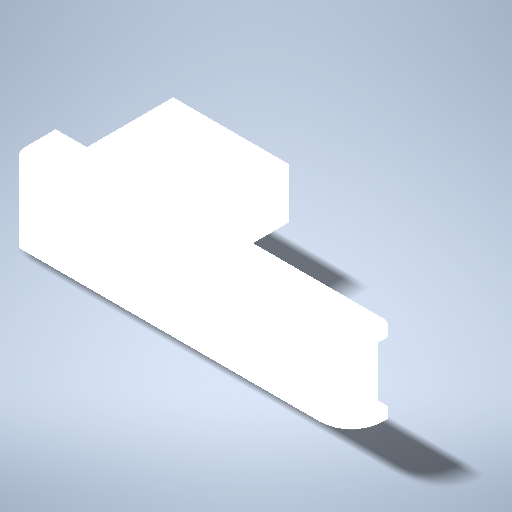
# Autodesk Inventor part: stereotax_holder_side
Saved by Autodesk Inventor 2025 (Build 290162000, 162)
## iProperties
Created: 2023-10-03
Part Number: stereotax_holder_side
Material: Generic
Document SubType Name: Modeling
Designer: mmelin
Density: 1 g/cm^3
Appearance: Default
Author: mmelin
Autodesk Inventor part; units mm, degrees
ref_plane "YZ Plane" through (0, 0, 0) normal (1, 0, 0) x (0, 1, 0)
ref_plane "XZ Plane" through (0, 0, 0) normal (0, 1, 0) x (-1, 0, 0)
ref_plane "XY Plane" through (0, 0, 0) normal (0, 0, 1) x (1, 0, 0)
sketch "Sketch1" plane through (0, 0, 0) normal (0, 0, 1) x (1, 0, 0)
  line L0 (-6.6, -4.4) -> (-23.2373, -4.4) projected
  line L1 (-23.2373, 1) -> (-6.6, 1) projected
  line L2 (-4.6226, -4.4) -> (-25.2226, -4.4)
  line L3 (-25.2226, -4.4) -> (-25.2226, 1)
  line L4 (-25.2226, 1) -> (-4.6226, 1)
  line L5 (-4.6226, 1) -> (-4.6226, -4.4)
  line L6 (-11.6, -0.9) -> (-11.6, -3.4) projected
  line L7 (-4.6226, 0.16) -> (-4.6226, -3.56) projected
  line L8 (-4.6226, 0.16) -> (-15, 0.16) projected
  line L9 (-15, 0.16) -> (-15, -3.56) projected
  line L10 (-15, -3.56) -> (-4.6226, -3.56) projected
  point P0 (0, 0)
  dimension "d1" = 20.6
  dimension "d36" = 0
  constraints: 8 end point, 2 collinear, 2 parallel, 1 horizontal, 1 perpendicular
  measures "d1" distance between parallel lines of L3 L5
  measures "d36" distance between parallel lines of L7 L5
extrude "Extrusion1" add sketch "Sketch1" along normal blind 1.7
sketch "Sketch2" plane through (0, 0, 0) normal (0, 0, -1) x (-1, 0, 0)
  line L0 (4.6226, 0.16) -> (4.6226, -3.56) projected
  line L1 (4.6226, 0.16) -> (15, 0.16) projected
  line L2 (15, 0.16) -> (15, -3.56) projected
  line L3 (15, -3.56) -> (4.6226, -3.56) projected
  line L4 (25.2226, -4.4) -> (4.6226, -4.4) projected
  line L5 (25.2226, 1) -> (25.2226, -4.4) projected
  line L6 (8.5501, -0.0891) -> (8.5501, -3.1391) projected
  line L7 (25.2226, -4.4) -> (4.6226, -4.4) projected
  line L8 (4.6226, -4.4) -> (4.6226, 1) projected
  line L9 (4.6226, 1) -> (25.2226, 1) projected
  line L10 (25.2226, 1) -> (25.2226, -4.4) projected
  line L11 (11.8, -2.35) -> (15, -2.35) projected
  line L12 (11.8, -1.05) -> (11.8, -2.35) projected
  line L13 (15, -1.05) -> (11.8, -1.05) projected
  point P0 (0, 0)
extrude "Extrusion2" add sketch "Sketch2" along normal blind 0.6 contours L8 L9 L5 L4 L3 L2 L1 | L2 L11 L12 L13
fillet "Fillet1" radius 2 1 edges at (-4.6226, -1.7, 1.7)
sketch "Sketch4" plane through (0, 0, -0.6) normal (0, 0, -1) x (-1, 0, 0)
  line L0 (24.45, -3.25) -> (17.25, -3.25)
  line L1 (17.25, -3.25) -> (17.25, -0.15)
  line L2 (17.25, -0.15) -> (24.45, -0.15)
  line L3 (24.45, -0.15) -> (24.45, -3.25)
  line L4 (24.6, -3.4) -> (24.6, 0) projected
  line L5 (17.1, -3.4) -> (24.6, -3.4) projected
  line L6 (17.1, 0) -> (17.1, -3.4) projected
  line L7 (24.6, 0) -> (17.1, 0) projected
  circle A0 centre (20.85, -1.7) radius 1.1 projected
  circle A1 centre (20.85, -1.7) radius 1.1
  point P0 (0, 0)
  dimension "d14" = 0.15
  dimension "d15" = 0.15
  dimension "d16" = 0.15
  dimension "d17" = 0.15
  constraints: 8 end point, 2 parallel, 1 centre point, 1 coincident, 1 concentric, 1 horizontal, 1 perpendicular
  measures "d14" distance between parallel lines of L7 L2
  measures "d15" distance between parallel lines of L6 L1
  measures "d16" distance between parallel lines of L4 L3
  measures "d17" distance between parallel lines of L5 L0
extrude "Extrusion5" add sketch "Sketch4" along normal blind 6.5 contours L0 L1 L2 L3
sketch "Sketch6" plane through (0, 0, 1.7) normal (0, 0, 1) x (1, 0, 0)
  circle A0 centre (-20.85, -1.7) radius 1.1 projected
  circle A1 centre (-20.85, -1.7) radius 1.1
  point P0 (0, 0)
  constraints: 1 centre point, 1 coincident
extrude "Extrusion7" cut sketch "Sketch6" against normal up to surface (8.8 mm away)
sketch "Sketch7" plane through (0, 0, 1.7) normal (0, 0, 1) x (1, 0, 0)
  circle A0 centre (-20.85, -1.7) radius 1.1 projected
  line L0 (-18.9, -2.8258) -> (-20.85, -3.9517)
  line L1 (-20.85, -3.9517) -> (-22.8, -2.8258)
  line L2 (-22.8, -2.8258) -> (-22.8, -0.5742)
  line L3 (-22.8, -0.5742) -> (-20.85, 0.5517)
  line L4 (-20.85, 0.5517) -> (-18.9, -0.5742)
  line L5 (-18.9, -0.5742) -> (-18.9, -2.8258)
  point P0 (0, 0)
  dimension "d27" = 3.9
  constraints: 12 end point, 1 coincident, 1 vertical, 13 other
  measures "d27" distance between parallel lines of L5 L2
extrude "Extrusion8" cut sketch "Sketch7" against normal blind 1.5
fillet "Fillet2" radius 0.3 6 edges at (-15.9226, 1, 1.7) (-5.2084, 1, 1.1142) (-4.6226, 1, -0.45) (-15.9226, -4.4, 1.7) (-5.2084, -4.4, 1.1142) (-4.6226, -4.4, -0.45)
equation "\"d15\" = d14"
equation "\"d16\" = d14"
equation "\"d17\" = d14"
body "Solid1"
